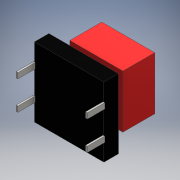
# Autodesk Inventor part: NINIGI_TACTS-24N
Saved by Autodesk Inventor 2016 (Build 200138000, 138)
## iProperties
Created: 2018-08-01
Part Number: NINIGI_TACTS-24N
Material: Generic
Document SubType Name: Modeling
Designer: Luke
Density: 1 g/cm^3
Appearance: Default
Author: Luke
Autodesk Inventor part; units mm, degrees
ref_plane "YZ Plane" through (0, 0, 0) normal (1, 0, 0) x (0, 1, 0)
ref_plane "XZ Plane" through (0, 0, 0) normal (0, 1, 0) x (-1, 0, 0)
ref_plane "XY Plane" through (0, 0, 0) normal (0, 0, 1) x (1, 0, 0)
sketch "Sketch1" plane through (0, 0, 0) normal (0, 1, 0) x (-1, 0, 0)
  line L0 (-0.15, 0.475) -> (0.15, 0.475)
  line L1 (0.15, 0.475) -> (0.15, -0.475)
  line L2 (0.15, -0.475) -> (-0.15, -0.475)
  line L3 (-0.15, -0.475) -> (-0.15, 0.475)
  line L4 (-0.15, 0.475) -> (0.15, -0.475) construction
  line L5 (0.15, 0.475) -> (-0.15, -0.475) construction
  line L6 (-0.15, 5.475) -> (0.15, 5.475)
  line L7 (0.15, 5.475) -> (0.15, 4.525)
  line L8 (0.15, 4.525) -> (-0.15, 4.525)
  line L9 (-0.15, 4.525) -> (-0.15, 5.475)
  line L10 (-0.15, 5.475) -> (0.15, 4.525) construction
  line L11 (0.15, 5.475) -> (-0.15, 4.525) construction
  line L12 (0, -1.665) -> (0, 6.665) construction
  line L13 (-14.61, 0) -> (2.61, 0) construction
  line L14 (-12.15, 0.475) -> (-11.85, 0.475)
  line L15 (-11.85, 0.475) -> (-11.85, -0.475)
  line L16 (-11.85, -0.475) -> (-12.15, -0.475)
  line L17 (-12.15, -0.475) -> (-12.15, 0.475)
  line L18 (-12.15, 0.475) -> (-11.85, -0.475) construction
  line L19 (-11.85, 0.475) -> (-12.15, -0.475) construction
  line L20 (-12.15, 5.475) -> (-11.85, 5.475)
  line L21 (-11.85, 5.475) -> (-11.85, 4.525)
  line L22 (-11.85, 4.525) -> (-12.15, 4.525)
  line L23 (-12.15, 4.525) -> (-12.15, 5.475)
  line L24 (-12.15, 5.475) -> (-11.85, 4.525) construction
  line L25 (-11.85, 5.475) -> (-12.15, 4.525) construction
  line L26 (-12, 0) -> (-12, 5) construction
  line L27 (-12, 5) -> (0, 5) construction
  point P0 (0, 0)
  point P1 (0, 5)
  point P2 (-12, 0)
  dimension "d0" = 0.95
  dimension "d1" = 0.3
  dimension "d2" = 0.95
  dimension "d3" = 0.3
  dimension "d4" = 5
  dimension "d5" = 0.95
  dimension "d6" = 0.3
  dimension "d7" = 12
  dimension "d8" = 0.95
  dimension "d9" = 0.3
  constraints: 52 end point, 10 midpoint, 10 parallel, 4 horizontal, 4 perpendicular, 2 point on line
  measures "d0" distance of L0.end L1.end
  measures "d1" distance of L1.end L2.end
  measures "d2" distance of L6.end L7.end
  measures "d3" distance of L7.end L8.end
  measures "d4" distance of point (0, 5) point (0, 0)
  measures "d5" distance of L14.end L15.end
  measures "d6" distance of L15.end L16.end
  measures "d7" distance of point (0, 0) point (-12, 0)
  measures "d8" distance of L20.end L21.end
  measures "d9" distance of L21.end L22.end
extrude "Extrusion1" add sketch "Sketch1" against normal blind 3
sketch "Sketch2" plane through (0, 0, 0) normal (0, 1, 0) x (-1, 0, 0)
  line L0 (0, -3.5) -> (-12, -3.5)
  line L1 (-12, -3.5) -> (-12, 8.5)
  line L2 (-12, 8.5) -> (0, 8.5)
  line L3 (0, 8.5) -> (0, -3.5)
  line L4 (0, -3.5) -> (-12, 8.5) construction
  line L5 (0, 8.5) -> (-12, -3.5) construction
  line L6 (-12.15, 5.475) -> (-11.85, 5.475) construction
  line L7 (-12.15, 4.525) -> (-12.15, 5.475) construction
  line L8 (-11.85, 4.525) -> (-12.15, 4.525) construction
  line L9 (-11.85, 5.475) -> (-11.85, 4.525) construction
  line L10 (-11.85, 5.475) -> (-11.85, 4.525) construction
  line L11 (-11.85, 5) -> (-12.15, 5) construction
  point P0 (0, 0)
  point P1 (-6, 2.5)
  point P2 (-6, 2.5)
  dimension "d12" = 12
  dimension "d13" = 12
  dimension "d14" = 6
  dimension "d15" = 2.5
  constraints: 14 end point, 3 midpoint, 2 parallel, 1 coincident, 1 horizontal, 1 perpendicular
  measures "d12" distance of L0.start L0.end
  measures "d13" distance of L0.end L1.end
  measures "d14" horizontal distance of point (-6, 2.5) point (0, 0)
  measures "d15" vertical distance of point (-6, 2.5) point (0, 0)
extrude "Extrusion2" add sketch "Sketch2" along normal blind 2.5
sketch "Sketch3" plane through (0, 2.5, 0) normal (0, 1, 0) x (1, 0, 0)
  line L0 (12, 3.5) -> (0, 3.5) construction
  line L1 (0, 3.5) -> (0, -8.5) construction
  line L2 (0, -8.5) -> (12, -8.5) construction
  line L3 (12, -8.5) -> (12, 3.5) construction
  line L4 (0, 3.5) -> (12, 3.5) construction
  line L5 (0, 3.5) -> (12, -8.5) construction
  line L6 (12, -8.5) -> (0, -8.5) construction
  line L7 (0, -8.5) -> (12, 3.5) construction
  circle A0 centre (6, -2.5) radius 3.35
  point P0 (0, 0)
  dimension "d18" = 6.7
  constraints: 4 end point, 1 centre point, 1 midpoint, 1 perpendicular
  measures "d18" diameter of A0
extrude "Extrusion3" add sketch "Sketch3" along normal blind 1
sketch "Sketch4" plane through (6, 3.5, 2.5) normal (0, 1, 0) x (1, 0, 0)
  circle A0 centre (0, 0) radius 3.35 projected
  line L0 (-3, -3) -> (3, -3)
  line L1 (3, -3) -> (3, 3)
  line L2 (3, 3) -> (-3, 3)
  line L3 (-3, 3) -> (-3, -3)
  line L4 (-3, -3) -> (3, 3) construction
  line L5 (3, -3) -> (-3, 3) construction
  point P0 (-6, 2.5)
  dimension "d21" = 6
  dimension "d22" = 6
  constraints: 12 end point, 2 midpoint, 2 parallel, 1 horizontal, 1 perpendicular
  measures "d21" distance of L0.end L1.end
  measures "d22" distance of L1.end L2.end
extrude "Extrusion4" add sketch "Sketch4" along normal blind 1.2 contours L1 A0 L0 L3 L2 | A0 L2 L1 | L1 L0 A0 | A0 L3 L2 | L0 L3 A0
sketch "Sketch5" plane through (6, 4.7, 2.5) normal (0, 1, 0) x (1, 0, 0)
  circle A0 centre (0, 0) radius 3.35 construction
  line L0 (6, 6) -> (-6, 6) construction
  line L1 (-6, 6) -> (-6, -6) construction
  line L2 (-6, -6) -> (6, -6) construction
  line L3 (6, -6) -> (6, 6) construction
  line L4 (-4.575, -4.575) -> (4.575, -4.575)
  line L5 (4.575, -4.575) -> (4.575, 4.575)
  line L6 (4.575, 4.575) -> (-4.575, 4.575)
  line L7 (-4.575, 4.575) -> (-4.575, -4.575)
  line L8 (-4.575, -4.575) -> (4.575, 4.575) construction
  line L9 (4.575, -4.575) -> (-4.575, 4.575) construction
  point P0 (-6, 2.5)
  dimension "d25" = 9.15
  dimension "d26" = 9.15
  constraints: 12 end point, 2 midpoint, 2 parallel, 1 horizontal, 1 perpendicular
  measures "d25" distance of L4.end L5.end
  measures "d26" distance of L5.end L6.end
extrude "Extrusion5" add sketch "Sketch5" along normal blind 5.5
equation "\"d13\" = d12"
equation "\"d22\" = d21"
equation "\"d26\" = d25"
body "Solid1"
